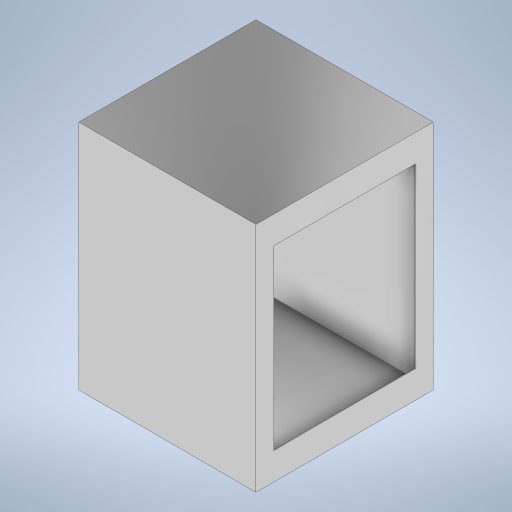
# Autodesk Inventor part: ASTRA_Body
Saved by Autodesk Inventor 2023.2 (Build 272271030, 271C)
## iProperties
Created: 2023-04-10
Part Number: ASTRA_Body
Material: Aluminum 6061
Document SubType Name: Modeling
Designer: ckeer
Density: 2.7 g/cm^3
Appearance: Chrome - Polished
Mass: 222132 g
Surface Area: 259822 cm^2
Volume: 82271.3 cm^3
Author: ckeer
Autodesk Inventor part; units mm, degrees
ref_plane "YZ Plane" through (0, 0, 0) normal (1, 0, 0) x (0, 1, 0)
ref_plane "XZ Plane" through (0, 0, 0) normal (0, 1, 0) x (-1, 0, 0)
ref_plane "XY Plane" through (0, 0, 0) normal (0, 0, 1) x (1, 0, 0)
sketch "Sketch1" plane through (0, 0, 0) normal (0, 1, 0) x (-1, 0, 0)
  line L0 (0, 0) -> (1524, 0)
  line L1 (1524, 0) -> (1524, -1524)
  line L2 (1524, -1524) -> (0, -1524)
  line L3 (0, -1524) -> (0, 0)
  line L4 (1517.65, -1517.65) -> (6.35, -1517.65)
  line L5 (6.35, -1517.65) -> (6.35, -6.35)
  line L6 (6.35, -6.35) -> (1517.65, -6.35)
  line L7 (1517.65, -6.35) -> (1517.65, -1517.65)
  dimension "d0" = 1524
  dimension "d1" = 1524
  dimension "d4" = 6.35
  dimension "d5" = 6.35
  dimension "d6" = 6.35
  dimension "d7" = 6.35
  constraints: 16 end point, 4 parallel, 2 horizontal, 2 perpendicular
  measures "d0" distance of L0.end L1.end
  measures "d1" distance of L1.end L2.end
  measures "d4" distance between parallel lines of L1 L7
  measures "d5" distance between parallel lines of L0 L6
  measures "d6" distance between parallel lines of L3 L5
  measures "d7" distance between parallel lines of L2 L4
extrude "Extrusion2" add sketch "Sketch1" along normal blind 1981.2
sketch "Sketch2" plane through (0, 1981.2, 0) normal (0, 1, 0) x (1, 0, 0)
  line L0 (0, 1524) -> (-1524, 1524) projected
  line L1 (0, 0) -> (-1524, 0)
  line L2 (-1524, 0) -> (-1524, 1524)
  line L3 (-1524, 1524) -> (0, 1524)
  line L4 (0, 1524) -> (0, 0)
  constraints: 8 end point, 2 parallel, 1 horizontal, 1 perpendicular
extrude "Extrusion3" add sketch "Sketch2" along normal blind 6.35
sketch "Sketch3" plane through (0, 0, 0) normal (0, -1, 0) x (1, 0, 0)
  line L0 (0, 0) -> (0, -1524) projected
  line L1 (0, -1524) -> (-1524, -1524) projected
  line L2 (0, 0) -> (-1524, 0)
  line L3 (-1524, 0) -> (-1524, -1524)
  line L4 (-1524, -1524) -> (0, -1524)
  line L5 (0, -1524) -> (0, 0)
  constraints: 8 end point, 2 parallel, 1 horizontal, 1 perpendicular
extrude "Extrusion4" add sketch "Sketch3" along normal blind 6.35
sketch "Sketch5" plane through (-1524, 1987.55, -1524) normal (-1, 0, 0) x (0, 0, 1)
  line L0 (1371.6, -234.95) -> (152.4, -234.95)
  line L1 (152.4, -234.95) -> (152.4, -1758.95)
  line L2 (152.4, -1758.95) -> (1371.6, -1758.95)
  line L3 (1371.6, -1758.95) -> (1371.6, -234.95)
  line L4 (1524, -1993.9) -> (1524, 0) projected
  line L5 (1524, -1993.9) -> (0, -1993.9) projected
  point P0 (1524, -1987.55)
  dimension "d21" = 1219.2
  dimension "d22" = 1524
  dimension "d23" = 152.4
  dimension "d24" = 234.95
  constraints: 8 end point, 2 parallel, 1 horizontal, 1 perpendicular
  measures "d21" distance of L0.start L0.end
  measures "d22" distance of L2.end L0.start
  measures "d23" distance between parallel lines of L4 L3
  measures "d24" distance between parallel lines of L5 L2
extrude "Extrusion6" cut sketch "Sketch5" against normal through all
body "Solid2"
